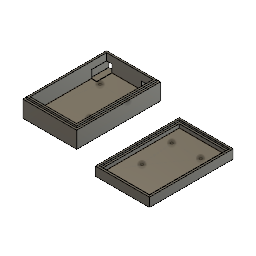
BME590lightbox v6 (Autodesk Fusion 360 design; units mm, degrees)
Autodesk Fusion 360 part; units mm, degrees
sketch "Sketch1" plane through (0, 0, 0) normal (0, 1, 0) x (1, 0, 0)
  line L0 (36.83, 57.15) -> (-36.83, 57.15)
  line L1 (-36.83, 57.15) -> (-36.83, -57.15)
  line L2 (-36.83, -57.15) -> (36.83, -57.15)
  line L3 (36.83, -57.15) -> (36.83, 57.15)
  line L4 (36.83, 57.15) -> (-36.83, -57.15) construction
  line L5 (-36.83, 57.15) -> (36.83, -57.15) construction
  dimension "d1" = 114.3
  dimension "d2" = 73.66
extrude "Extrude1" add sketch "Sketch1" along normal blind 25.4 makes body 1
shell "Shell1" thickness 5.08 removed faces 1 at (12.2767, 25.4, 19.05) on bodies 1
sketch "Sketch4" plane through (0, 25.4, 0) normal (0, 1, 0) x (-1, 0, 0)
  line L0 (-31.75, 52.07) -> (31.75, 52.07)
  line L1 (31.75, 52.07) -> (31.75, -52.07)
  line L2 (31.75, -52.07) -> (-31.75, -52.07)
  line L3 (-31.75, -52.07) -> (-31.75, 52.07)
  line L4 (-36.83, 57.15) -> (-36.83, -57.15)
  line L5 (-36.83, -57.15) -> (36.83, -57.15)
  line L6 (36.83, -57.15) -> (36.83, 57.15)
  line L7 (36.83, 57.15) -> (-36.83, 57.15)
  line L8 (34.29, 54.61) -> (-34.29, 54.61)
  line L9 (-34.29, 54.61) -> (-34.29, -54.61)
  line L10 (-34.29, -54.61) -> (34.29, -54.61)
  line L11 (34.29, -54.61) -> (34.29, 54.61)
  dimension "d8" = 2.54
extrude "Extrude2" cut sketch "Sketch4" against normal blind 2.54 contours L4 L5 L6 L7 bodies 1
sketch "Sketch5" plane through (0, 0, 0) normal (0, 1, 0) x (1, 0, 0)
  line L0 (30.48, 38.1) -> (104.14, 38.1)
  line L1 (104.14, 38.1) -> (104.14, -76.2)
  line L2 (104.14, -76.2) -> (30.48, -76.2)
  line L3 (30.48, -76.2) -> (30.48, 38.1)
  dimension "d11" = 73.66
  dimension "d12" = 114.3
extrude "Extrude3" add sketch "Sketch5" along normal blind 10.16 separate body makes body 2
shell "Shell2" thickness 5.08 removed faces 1 at (55.0333, 10.16, 0) on bodies 2
sketch "Sketch6" plane through (0, 10.16, 0) normal (0, 1, 0) x (-1, 0, 0)
  line L0 (-35.56, 71.12) -> (-35.56, -33.02)
  line L1 (-35.56, -33.02) -> (-99.06, -33.02)
  line L2 (-99.06, -33.02) -> (-99.06, 71.12)
  line L3 (-99.06, 71.12) -> (-35.56, 71.12)
  line L4 (-30.48, 76.2) -> (-104.14, 76.2)
  line L5 (-104.14, 76.2) -> (-104.14, -38.1)
  line L6 (-104.14, -38.1) -> (-30.48, -38.1)
  line L7 (-30.48, -38.1) -> (-30.48, 76.2)
  line L8 (-33.02, 73.66) -> (-101.6, 73.66)
  line L9 (-101.6, 73.66) -> (-101.6, -35.56)
  line L10 (-101.6, -35.56) -> (-33.02, -35.56)
  line L11 (-33.02, -35.56) -> (-33.02, 73.66)
  dimension "d16" = 2.54
extrude "Extrude4" add sketch "Sketch6" along normal blind 2.286 contours L4 L5 L6 L7 bodies 2
move_body "Move1" bodies 2 to x (1, 0, 0) y (0, 1, 0) z (0, 0, 1) at (50.8, 0, 0)
sketch "Sketch7" plane through (0, 5.08, 0) normal (0, 1, 0) x (-1, 0, 0)
  line L0 (-31.75, 52.07) -> (-31.75, -52.07)
  line L1 (-31.75, -52.07) -> (31.75, -52.07)
  line L2 (31.75, -52.07) -> (31.75, 52.07)
  line L3 (31.75, 52.07) -> (-31.75, 52.07)
  circle A0 centre (19.05, -30.48) radius 1.6002
  circle A1 centre (-19.05, -29.21) radius 1.6002
  circle A2 centre (-13.97, 16.51) radius 1.6002
  dimension "d19" = 3.2004
  dimension "d21" = 12.7
  dimension "d22" = 21.59
  dimension "d23" = 3.2004
  dimension "d24" = 12.7
  dimension "d25" = 22.86
  dimension "d26" = 3.2004
  dimension "d27" = 45.72
  dimension "d28" = 35.56
  measures "d19" diameter of A0
  measures "d23" diameter of A1
  measures "d26" diameter of A2
sketch "Sketch8" plane through (0, 5.08, 0) normal (0, 1, 0) x (-1, 0, 0)
  line L0 (-86.36, 71.12) -> (-149.86, 71.12)
  line L1 (-149.86, 71.12) -> (-149.86, -33.02)
  line L2 (-149.86, -33.02) -> (-86.36, -33.02)
  line L3 (-86.36, -33.02) -> (-86.36, 71.12)
  circle A0 centre (-137.16, -11.43) radius 1.6002
  circle A1 centre (-99.06, -10.16) radius 1.6002
  circle A2 centre (-104.14, 35.56) radius 1.6002
  dimension "d29" = 3.2004
  dimension "d30" = 12.7
  dimension "d31" = 21.59
  dimension "d32" = 3.2004
  dimension "d33" = 12.7
  dimension "d34" = 22.86
  dimension "d35" = 3.2004
  dimension "d36" = 45.72
  dimension "d37" = 35.56
  measures "d29" diameter of A0
  measures "d32" diameter of A1
  measures "d35" diameter of A2
sketch "Sketch9" plane through (0, 0, -57.15) normal (0, 0, -1) x (-1, 0, 0)
  line L0 (36.83, 22.86) -> (-36.83, 22.86)
  line L1 (-36.83, 22.86) -> (-36.83, 0)
  line L2 (-36.83, 0) -> (36.83, 0)
  line L3 (36.83, 0) -> (36.83, 22.86)
  line L4 (33.655, 4.572) -> (24.765, 4.572)
  line L5 (24.765, 4.572) -> (24.765, 15.621)
  line L6 (24.765, 15.621) -> (33.655, 15.621)
  line L7 (33.655, 15.621) -> (33.655, 4.572)
  line L8 (33.655, 4.572) -> (24.765, 15.621) construction
  line L9 (24.765, 4.572) -> (33.655, 15.621) construction
  line L10 (-15.875, 15.621) -> (-27.305, 15.621)
  line L11 (-27.305, 15.621) -> (-27.305, 4.826)
  line L12 (-27.305, 4.826) -> (-15.875, 4.826)
  line L13 (-15.875, 4.826) -> (-15.875, 15.621)
  line L14 (-15.875, 15.621) -> (-27.305, 4.826) construction
  line L15 (-27.305, 15.621) -> (-15.875, 4.826) construction
  dimension "d38" = 8.89
  dimension "d39" = 11.049
  dimension "d40" = 3.175
  dimension "d42" = 18.288
  dimension "d43" = 11.43
  dimension "d44" = 10.795
  dimension "d45" = 9.525
  dimension "d46" = 7.239
  measures "d40" distance of L3 L7
  measures "d42" distance of L0 L4
  measures "d45" distance of L1 L11
  measures "d46" distance of L0 L10
extrude "Extrude5" cut sketch "Sketch9" against normal blind 25.4 contours L4 L5 L6 L7 bodies 1
sketch "Sketch10" plane through (0, 0, -57.15) normal (0, 0, -1) x (-1, 0, 0)
  line L0 (24.765, 4.572) -> (24.765, 15.621)
  line L1 (24.765, 15.621) -> (33.655, 15.621)
  line L2 (33.655, 15.621) -> (33.655, 4.572)
  line L3 (33.655, 4.572) -> (24.765, 4.572)
  line L4 (36.83, 22.86) -> (-36.83, 22.86)
  line L5 (-36.83, 22.86) -> (-36.83, 0)
  line L6 (-36.83, 0) -> (36.83, 0)
  line L7 (36.83, 0) -> (36.83, 22.86)
  line L8 (-15.875, 15.621) -> (-27.305, 15.621)
  line L9 (-27.305, 15.621) -> (-27.305, 4.826)
  line L10 (-27.305, 4.826) -> (-15.875, 4.826)
  line L11 (-15.875, 4.826) -> (-15.875, 15.621)
  line L12 (-15.875, 15.621) -> (-27.305, 4.826) construction
  line L13 (-27.305, 15.621) -> (-15.875, 4.826) construction
  dimension "d49" = 11.43
  dimension "d50" = 10.795
  dimension "d51" = 7.239
  dimension "d52" = 9.525
  measures "d51" distance of L4 L8
  measures "d52" distance of L5 L9
extrude "Extrude6" cut sketch "Sketch10" against normal blind 25.4 contours L8 L9 L10 L11 bodies 1
